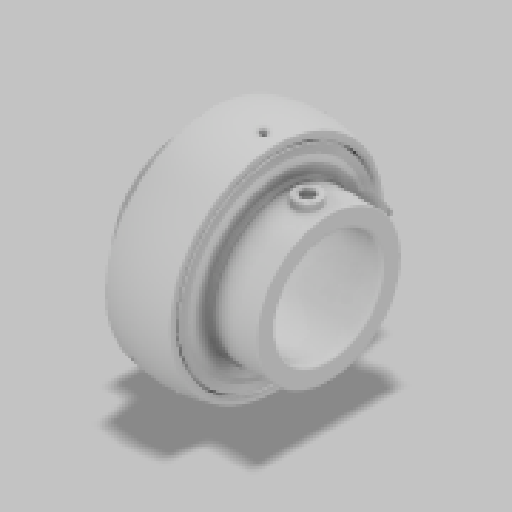
# Autodesk Inventor part: UC 205+33.7_b
Saved by Autodesk Inventor 2025.2 (Build 292293000, 293)
## iProperties
Category: PARTsolutions
Company: SKF
Created: 2024-04-15
Part Number: UC 205+33.7_b
Material: Generic
Catalog Web Link: www.cadenas.de
Description: ayf_002hc_hh_hy_ayd_001hp_b-Y-bearings
Vendor: SKF
Document SubType Name: Modeling
Designer: psAdmin
Manufacturer: SKF
Mass: 22.2114 g
Surface Area: 223.457 cm^2
Volume: 22.2114 cm^3
Density: 1 g/cm^3
Appearance: PSOLRGB-175-175-175
PSOL_IDENT_0: {$CADENAS_DATA/23d-libs/skf/bearings_units_and_housings/bearing_units/ball_bearing_units/y-units/y-b
PSOL_IDENT_1: earing_oval_flanged_units_parts/ayf_002hc_hh_hy_ayd_001hp_bearing.prj},189 {VTYP=3D},{NB=UC 205+33.7
PSOL_IDENT_2: _b},{LINA=UC 205+33.7_b},{NN=ayf_002hc_hh_hy_ayd_001hp_b},{DATE=28.11.2022 11:15:06},{GEOMDATE=25.11
PSOL_IDENT_3: .2022 07:55:51},{VERSION=},{LINEID=4060},{WBVAR=},{WBNUMERIC=}  {NB=UC 205+33.7_b},{LINA=UC 205+33.7
PSOL_IDENT_4: _b},{KT=DUMMY},{PRODUCTID=0},{DESIGNATION=UC 205},{DD=25.0000},{D=52},{B=34.000},{C=15.000},{PITCH=3
PSOL_IDENT_5: 9.000},{DW=7.938},{FO=IEC_BBY_006},{DESIGN=ucfl},{B1=34.000},{LM=},{DES=},{PS=},{MAT=},{SS=},{UNIT=}
PSOL_IDENT_6: ,{G=MIN},{DD1=33.70},{DD2=MIN},{DD3=MIN},{B3=0},{B4=5.5},{BB4=5.0},{R12=0.6},{R12X=0},{SS1=19.700},{
PSOL_IDENT_7: NOTE=},{DG=MIN},{E=4.350},{F=1.700},{RG=0.000},{LOAD1=14.000},{LOAD2=7.800},{LOAD3=0.335},{SPEED2=70
PSOL_IDENT_8: 00},{FF0=14},{BF=1},{A15=500000},{A8=400000},{A4=300000},{BETA=1.89},{SBT1=0.094},{SBT2=},{RF1=0.000
PSOL_IDENT_9: 00039},{RF2=1.7},{SF1=0.00323},{SF2=36.5},{KZ=3.1},{II=1},{Z=9},{SG=VT307},{MASS=0.19},{G2=M6x0.75},
PSOL_IDENT_10: {HEX=3.000},{RTT=4},{MKIT=},{AS=},{TANGLE=},{SLEEVE=},{SRING=RIS 205},{FPC=RBC17_YBRG_001},{POPI=1},
PSOL_IDENT_11: {NOUN=N020},{NOUNDES=Ball bearing},{MOD=M200},{MODDES=Radial deep groove},{YZ=16.85},{PIM=UCFL 205},
PSOL_IDENT_12: {LNDD11=MIN},{LUB3=0},{BZ=0.4708},{SDALG=h},{YRZ=23.469},{SHAPE=4},{LNB1HM11=0},{LWM=0},{TYPEID=0},{
PSOL_IDENT_13: LUBGR2=0},{LOCKNUT=},{LOCKDEVICE=},{LNB=MIN},{BB=MIN},{LNB1=MIN},{S1ALG=19.7},{HH=MIN},{LDB=MIN},{LD
PSOL_IDENT_14: DD1=MIN},{LDDD2=MIN},{LDM=MIN},{LDFF=MIN},{TP=4},{LNBHM11=0},{BBHM11=0},{LNDD1HM11=0},{HELP=5},{HHHM
PSOL_IDENT_15: 11=0},{LUBGR1=0},{LWV=0},{S2=25.9},{LUB2=1},{BZ1=0.000},{HEX2=},{B3A=0.000},{SS1ALG=19.700}
NB: UC 205+33.7_b
NN: ayf_002hc_hh_hy_ayd_001hp_b
NT: Y-bearings
NBSYN: $DESIGNATION.+$DD1._b
LINA: UC 205+33.7_b
CATALOG: SKF
DESIGNATION: UC 205
DD: 25
D: 52
B: 34
C: 15
PITCH: 39
DW: 7.938
FO: IEC_BBY_006
B1: 34
DD1: 33.7
LUB3: 0
SUPPLIER: SKF
ARTICLENO: UC 205+33.7_b
BOMINFO: UC 205+33.7_b
CREATOR: CADENAS GmbH
Title: UC 205+33.7_b
Author: Cadenas PARTsolutions
Comments: Y-bearings
Autodesk Inventor part; units mm, degrees
sketch "Sketch_35" plane through (0, 0, 0) normal (0, 0, 1) x (1, 0, 0)
  line L0 (50, 0) -> (-50, 0)
  line L1 (-14.3, 16.55) -> (-14.3, 13.1)
  arc A0 (-14.3, 13.1) -> (-13.7, 12.5) centre (-13.7, 13.1) ccw
  line L2 (-13.7, 12.5) -> (19.1, 12.5)
  arc A1 (19.1, 12.5) -> (19.7, 13.1) centre (19.1, 13.1) ccw
  line L3 (19.7, 13.1) -> (19.7, 16.55)
  arc A2 (19.7, 16.55) -> (19.4, 16.85) centre (19.4, 16.55) ccw
  line L4 (19.4, 16.85) -> (2.9547, 16.85)
  arc A3 (-2.9547, 16.85) -> (2.9547, 16.85) centre (0, 19.5) ccw
  line L5 (-2.9547, 16.85) -> (-14, 16.85)
  arc A4 (-14, 16.85) -> (-14.3, 16.55) centre (-14, 16.55) ccw
  constraints: 12 end point, 10 point on circle, 5 centre point
revolve "Revolution1" add sketch "Sketch_35" angle 360 about axis through (50, 0, 0) along (1, 0, 0)
sketch "Sketch_36" plane through (0, 12.5, 0) normal (0, 1, 0) x (1, 0, 0)
  circle A0 centre (14.7, 0) radius 3
  line L0 (13.2, -0.866) -> (14.7, -1.7321)
  line L1 (14.7, -1.7321) -> (16.2, -0.866)
  line L2 (16.2, -0.866) -> (16.2, 0.866)
  line L3 (16.2, 0.866) -> (14.7, 1.7321)
  line L4 (14.7, 1.7321) -> (13.2, 0.866)
  line L5 (13.2, 0.866) -> (13.2, -0.866)
  constraints: 12 end point, 1 centre point
extrude "Extrusion1" add sketch "Sketch_36" along normal blind 6
sketch "Sketch_37" plane through (0, 5.8684, -11.0368) normal (0, 0.4695, -0.8829) x (1, 0, 0)
  circle A0 centre (14.7, 0) radius 3
  line L0 (13.2, -0.866) -> (14.7, -1.7321)
  line L1 (14.7, -1.7321) -> (16.2, -0.866)
  line L2 (16.2, -0.866) -> (16.2, 0.866)
  line L3 (16.2, 0.866) -> (14.7, 1.7321)
  line L4 (14.7, 1.7321) -> (13.2, 0.866)
  line L5 (13.2, 0.866) -> (13.2, -0.866)
  constraints: 12 end point, 1 centre point
extrude "Extrusion2" add sketch "Sketch_37" along normal blind 6
sketch "Sketch_38" plane through (0, 0, 0) normal (0, 0, 1) x (1, 0, 0)
  line L0 (7.5, 0) -> (-7.5, 0)
  line L1 (-9.877, 17.3208) -> (-9.877, 16.85)
  line L2 (-9.877, 16.85) -> (-7.9938, 16.85)
  line L3 (-7.9938, 16.85) -> (-7.9938, 19.5)
  line L4 (-7.9938, 19.5) -> (-7.2646, 20.823)
  line L5 (-7.2646, 20.823) -> (-7.2646, 22.7336)
  line L6 (-7.2646, 22.7336) -> (-7.7354, 22.7336)
  line L7 (-7.7354, 22.7336) -> (-7.7354, 20.823)
  line L8 (-7.7354, 20.823) -> (-8.4646, 19.5)
  line L9 (-8.4646, 19.5) -> (-8.4646, 17.3208)
  line L10 (-8.4646, 17.3208) -> (-9.877, 17.3208)
  constraints: 22 end point
revolve "Revolution2" add sketch "Sketch_38" angle 360 about axis through (7.5, 0, 0) along (1, 0, 0)
sketch "Sketch_39" plane through (0, 0, 0) normal (0, 0, 1) x (1, 0, 0)
  line L0 (7.5, 0) -> (-7.5, 0)
  line L1 (7.2646, 22.7336) -> (7.2646, 20.823)
  line L2 (7.2646, 20.823) -> (7.9938, 19.5)
  line L3 (7.9938, 19.5) -> (7.9938, 16.85)
  line L4 (7.9938, 16.85) -> (9.877, 16.85)
  line L5 (9.877, 16.85) -> (9.877, 17.3208)
  line L6 (9.877, 17.3208) -> (8.4646, 17.3208)
  line L7 (8.4646, 17.3208) -> (8.4646, 19.5)
  line L8 (8.4646, 19.5) -> (7.7354, 20.823)
  line L9 (7.7354, 20.823) -> (7.7354, 22.7336)
  line L10 (7.7354, 22.7336) -> (7.2646, 22.7336)
  constraints: 22 end point
revolve "Revolution3" add sketch "Sketch_39" angle 360 about axis through (7.5, 0, 0) along (1, 0, 0)
sketch "Sketch_40" plane through (0, 0, 0) normal (0, 0, 1) x (1, 0, 0)
  line L0 (50, 0) -> (-50, 0)
  line L1 (-7.5, 19.9406) -> (-7.5, 17.2471)
  line L2 (-7.5, 17.2471) -> (-7.0292, 17.2471)
  line L3 (-7.0292, 17.2471) -> (-7.0292, 19.6938)
  line L4 (-7.0292, 19.6938) -> (-5.0717, 21.0482)
  line L5 (-5.0717, 21.0482) -> (-5.0181, 20.9708)
  line L6 (-5.0181, 20.9708) -> (-6.935, 19.6444)
  line L7 (-6.935, 19.6444) -> (-6.935, 17.4457)
  line L8 (-6.935, 17.4457) -> (-5.1617, 17.4457)
  line L9 (-5.1617, 17.4457) -> (-5.3029, 16.85)
  line L10 (-5.3029, 16.85) -> (-4.8321, 16.85)
  line L11 (-4.8321, 16.85) -> (-4.6752, 17.5119)
  line L12 (-4.6752, 17.5119) -> (-4.6752, 18.1738)
  line L13 (-4.6752, 18.1738) -> (-5.3029, 18.8357)
  line L14 (-5.3029, 18.8357) -> (-5.3029, 20.1595)
  line L15 (-5.3029, 20.1595) -> (-4.6752, 20.8214)
  line L16 (-4.6752, 20.8214) -> (-4.6752, 23.3121)
  arc A0 (-4.6752, 23.3121) -> (-4.8321, 23.469) centre (-4.8321, 23.3121) ccw
  line L17 (-4.8321, 23.469) -> (-4.9891, 23.469)
  arc A1 (-4.9891, 23.469) -> (-5.146, 23.3121) centre (-4.9891, 23.3121) ccw
  line L18 (-5.146, 23.3121) -> (-5.9775, 22.3212)
  line L19 (-5.9775, 22.3212) -> (-5.6168, 22.0186)
  line L20 (-5.6168, 22.0186) -> (-5.146, 22.5796)
  line L21 (-5.146, 22.5796) -> (-5.146, 21.5693)
  line L22 (-5.146, 21.5693) -> (-7.5, 19.9406)
  constraints: 46 end point, 4 point on circle, 2 centre point
revolve "Revolution4" add sketch "Sketch_40" angle 360 about axis through (50, 0, 0) along (1, 0, 0)
sketch "Sketch_41" plane through (0, 0, 0) normal (0, 0, 1) x (1, 0, 0)
  line L0 (50, 0) -> (-50, 0)
  line L1 (4.6752, 23.3121) -> (4.6752, 20.8214)
  line L2 (4.6752, 20.8214) -> (5.3029, 20.1595)
  line L3 (5.3029, 20.1595) -> (5.3029, 18.8357)
  line L4 (5.3029, 18.8357) -> (4.6752, 18.1738)
  line L5 (4.6752, 18.1738) -> (4.6752, 17.5119)
  line L6 (4.6752, 17.5119) -> (4.8321, 16.85)
  line L7 (4.8321, 16.85) -> (5.3029, 16.85)
  line L8 (5.3029, 16.85) -> (5.1617, 17.4457)
  line L9 (5.1617, 17.4457) -> (6.935, 17.4457)
  line L10 (6.935, 17.4457) -> (6.935, 19.6444)
  line L11 (6.935, 19.6444) -> (5.0181, 20.9708)
  line L12 (5.0181, 20.9708) -> (5.0717, 21.0482)
  line L13 (5.0717, 21.0482) -> (7.0292, 19.6938)
  line L14 (7.0292, 19.6938) -> (7.0292, 17.2471)
  line L15 (7.0292, 17.2471) -> (7.5, 17.2471)
  line L16 (7.5, 17.2471) -> (7.5, 19.9406)
  line L17 (7.5, 19.9406) -> (5.146, 21.5693)
  line L18 (5.146, 21.5693) -> (5.146, 22.5796)
  line L19 (5.146, 22.5796) -> (5.6168, 22.0186)
  line L20 (5.6168, 22.0186) -> (5.9775, 22.3212)
  line L21 (5.9775, 22.3212) -> (5.146, 23.3121)
  arc A0 (5.146, 23.3121) -> (4.9891, 23.469) centre (4.9891, 23.3121) ccw
  line L22 (4.9891, 23.469) -> (4.8321, 23.469)
  arc A1 (4.8321, 23.469) -> (4.6752, 23.3121) centre (4.8321, 23.3121) ccw
  constraints: 46 end point, 4 point on circle, 2 centre point
revolve "Revolution5" add sketch "Sketch_41" angle 360 about axis through (50, 0, 0) along (1, 0, 0)
sketch "Sketch_16" plane through (0, 0, 0) normal (0, 0, 1) x (1, 0, 0)
  line L0 (7.5, 0) -> (-7.5, 0)
  line L1 (-7.5, 23.2586) -> (-5.2395, 23.2586)
  line L2 (-5.2395, 23.2586) -> (-5.0722, 23.3999)
  arc A0 (-4.6666, 23.2648) -> (-5.0722, 23.3999) centre (-4.9106, 23.2086) ccw
  line L3 (-4.6666, 23.2648) -> (-4.5664, 22.8303)
  arc A1 (-4.5664, 22.8303) -> (-4.3715, 22.6752) centre (-4.3715, 22.8752) ccw
  line L4 (-4.3715, 22.6752) -> (-2.4646, 22.6752)
  arc A2 (-2.4646, 22.6752) -> (-2.3164, 22.7229) centre (-2.4646, 22.9292) ccw
  arc A3 (2.3164, 22.7229) -> (-2.3164, 22.7229) centre (0, 19.5) ccw
  arc A4 (2.3164, 22.7229) -> (2.4646, 22.6752) centre (2.4646, 22.9292) ccw
  line L5 (2.4646, 22.6752) -> (4.3715, 22.6752)
  arc A5 (4.3715, 22.6752) -> (4.5664, 22.8303) centre (4.3715, 22.8752) ccw
  line L6 (4.5664, 22.8303) -> (4.6666, 23.2648)
  arc A6 (5.0722, 23.3999) -> (4.6666, 23.2648) centre (4.9106, 23.2086) ccw
  line L7 (5.0722, 23.3999) -> (5.2395, 23.2586)
  line L8 (5.2395, 23.2586) -> (7.5, 23.2586)
  line L9 (7.5, 23.2586) -> (7.5, 24.7457)
  arc A7 (7.5, 24.7457) -> (7.3566, 24.9375) centre (7.3, 24.7457) ccw
  arc A8 (7.3566, 24.9375) -> (-7.3566, 24.9375) centre (0, 0) ccw
  arc A9 (-7.3566, 24.9375) -> (-7.5, 24.7457) centre (-7.3, 24.7457) ccw
  line L10 (-7.5, 24.7457) -> (-7.5, 23.2586)
  constraints: 22 end point, 20 point on circle, 10 centre point
revolve "Revolution6" add sketch "Sketch_16" angle 360 about axis through (7.5, 0, 0) along (1, 0, 0)
sketch "Sketch_42" plane through (0, 0, 0) normal (0, 0, 1) x (1, 0, 0)
  line L0 (4.4, 19.5) -> (4.4, 39)
  line L1 (4.4, 39) -> (5.25, 39)
  line L2 (5.25, 39) -> (5.25, 19.5)
  line L3 (5.25, 19.5) -> (4.4, 19.5)
  line L4 (4.4, 19.5) -> (4.4, 39)
  constraints: 10 end point
revolve "Revolution7" cut sketch "Sketch_42" angle 360 about axis through (4.4, 19.5, 0) along (0, -1, 0)
sketch "Sketch_43" plane through (0, 0, 0) normal (0, -0.866, -0.5) x (1, 0, 0)
  line L0 (-3.5562, 19.5) -> (-3.5562, 39)
  line L1 (-3.5562, 39) -> (-2.7062, 39)
  line L2 (-2.7062, 39) -> (-2.7062, 19.5)
  line L3 (-2.7062, 19.5) -> (-3.5562, 19.5)
  line L4 (-3.5562, 19.5) -> (-3.5562, 39)
  constraints: 10 end point
revolve "Revolution8" cut sketch "Sketch_43" angle 360 about axis through (-3.5562, -9.75, 16.8875) along (0, 0.5, -0.866)
ref_plane "ball_1_XY" through (0, 19.5, 0) normal (1, 0, 0) x (0, 0, -1)
ref_plane "ball_1_YZ" through (0, 19.5, 0) normal (0, 0, -1) x (0, 1, 0)
ref_plane "ball_1_ZX" through (0, 19.5, 0) normal (0, 1, 0) x (1, 0, 0)
ref_plane "ball_2_XY" through (0, 14.9379, 12.5344) normal (1, 0, 0) x (0, 0, -1)
ref_plane "ball_2_YZ" through (0, 14.9379, 12.5344) normal (0, 0, -1) x (0, 1, 0)
ref_plane "ball_2_ZX" through (0, 14.9379, 12.5344) normal (0, 1, 0) x (1, 0, 0)
ref_plane "ball_3_XY" through (0, 3.3861, 19.2038) normal (1, 0, 0) x (0, 0, -1)
ref_plane "ball_3_YZ" through (0, 3.3861, 19.2038) normal (0, 0, -1) x (0, 1, 0)
ref_plane "ball_3_ZX" through (0, 3.3861, 19.2038) normal (0, 1, 0) x (1, 0, 0)
ref_plane "ball_4_XY" through (0, -9.75, 16.8875) normal (1, 0, 0) x (0, 0, -1)
ref_plane "ball_4_YZ" through (0, -9.75, 16.8875) normal (0, 0, -1) x (0, 1, 0)
ref_plane "ball_4_ZX" through (0, -9.75, 16.8875) normal (0, 1, 0) x (1, 0, 0)
ref_plane "ball_5_XY" through (0, -18.324, 6.6694) normal (1, 0, 0) x (0, 0, -1)
ref_plane "ball_5_YZ" through (0, -18.324, 6.6694) normal (0, 0, -1) x (0, 1, 0)
ref_plane "ball_5_ZX" through (0, -18.324, 6.6694) normal (0, 1, 0) x (1, 0, 0)
ref_plane "ball_6_XY" through (0, -18.324, -6.6694) normal (1, 0, 0) x (0, 0, -1)
ref_plane "ball_6_YZ" through (0, -18.324, -6.6694) normal (0, 0, -1) x (0, 1, 0)
ref_plane "ball_6_ZX" through (0, -18.324, -6.6694) normal (0, 1, 0) x (1, 0, 0)
ref_plane "ball_7_XY" through (0, -9.75, -16.8875) normal (1, 0, 0) x (0, 0, -1)
ref_plane "ball_7_YZ" through (0, -9.75, -16.8875) normal (0, 0, -1) x (0, 1, 0)
ref_plane "ball_7_ZX" through (0, -9.75, -16.8875) normal (0, 1, 0) x (1, 0, 0)
ref_plane "ball_8_XY" through (0, 3.3861, -19.2038) normal (1, 0, 0) x (0, 0, -1)
ref_plane "ball_8_YZ" through (0, 3.3861, -19.2038) normal (0, 0, -1) x (0, 1, 0)
ref_plane "ball_8_ZX" through (0, 3.3861, -19.2038) normal (0, 1, 0) x (1, 0, 0)
ref_plane "ball_9_XY" through (0, 14.9379, -12.5344) normal (1, 0, 0) x (0, 0, -1)
ref_plane "ball_9_YZ" through (0, 14.9379, -12.5344) normal (0, 0, -1) x (0, 1, 0)
ref_plane "ball_9_ZX" through (0, 14.9379, -12.5344) normal (0, 1, 0) x (1, 0, 0)
ref_plane "brg_XY" through (19.7, 0, 0) normal (1, 0, 0) x (0, 0, -1)
ref_plane "brg_YZ" through (19.7, 0, 0) normal (0, 0, -1) x (0, 1, 0)
ref_plane "brg_ZX" through (19.7, 0, 0) normal (0, 1, 0) x (1, 0, 0)
body "Solid1"
